Support motor cam 2 (Autodesk Fusion 360 design; units mm, degrees)
Autodesk Fusion 360 part; units mm, degrees
sketch "Support moteur/Cam" plane through (0, 0, 0) normal (0, 0, 1) x (1, 0, 0)
  line L0 (-113.5546, -207.3984) -> (-130.3546, -207.3984)
  line L1 (-130.3546, -207.3984) -> (-135.6849, -205.7263)
  line L2 (-135.6849, -205.7263) -> (-141.4789, -211.9329)
  line L3 (-141.4789, -211.9329) -> (-141.6802, -212.3176)
  line L4 (-141.6802, -212.3176) -> (-141.6802, -223.1)
  line L5 (-113.5528, -238.7984) -> (-130.3528, -238.8003)
  line L6 (-130.3528, -238.8003) -> (-135.6829, -240.4729)
  line L7 (-141.4776, -234.267) -> (-141.679, -233.8823)
  line L8 (-141.679, -233.8823) -> (-141.6802, -223.1)
  line L9 (-135.6829, -240.4729) -> (-141.4776, -234.267)
  circle A0 centre (-136.6035, -217.4087) radius 0.75
  circle A1 centre (-118.6035, -217.4087) radius 0.75
  circle A2 centre (-136.6035, -228.9087) radius 0.75
  circle A3 centre (-118.6035, -228.9087) radius 0.75
  line L10 (-113.5546, -207.3984) -> (-113.5528, -238.7984)
  line L11 (-141.6802, -223.1) -> (-113.5537, -223.0984)
  point P0 (-136.6035, -217.4087)
  point P1 (-118.6035, -217.4087)
  point P2 (-118.6035, -228.9087)
  point P3 (-136.6035, -228.9087)
  dimension "d217" = 16.8
  dimension "d227" = 1.5
  dimension "d228" = 1.5
  dimension "d229" = 1.5
  dimension "d230" = 1.5
  constraint horizontal L0
  constraint vertical L4
  constraint coincident P0 A0.centre
  constraint coincident P1 A1.centre
  constraint coincident P3 A2.centre
  constraint coincident P2 A3.centre
  constraint midpoint L10 L11.end
  constraint perpendicular L10 L11
  measures "d217" distance of L0.start L0.end
  measures "d227" diameter of A0
  measures "d228" diameter of A1
  measures "d229" diameter of A2
  measures "d230" diameter of A3
ref_plane "WorkPlane9" through (0, 0, -10.8) normal (0, 0, 1) x (1, 0, 0)
sketch "Support moteur/Cam2" plane through (0, 0, -10.8) normal (0, 0, 1) x (1, 0, 0)
  line L0 (-113.5546, -236.9984) -> (-130.3974, -237.1164)
  line L1 (-130.3974, -237.1164) -> (-135.6833, -238.6066)
  line L2 (-135.6833, -238.6066) -> (-138.7984, -232.7391)
  line L3 (-138.7984, -223.0984) -> (-138.7984, -232.7391)
  line L4 (-138.7984, -223.0984) -> (-138.7984, -213.4577)
  line L5 (-135.6833, -207.5901) -> (-138.7984, -213.4577)
  line L6 (-130.3974, -209.0804) -> (-135.6833, -207.5901)
  line L7 (-113.5546, -209.1984) -> (-130.3974, -209.0804)
  line L8 (-122.1546, -237.0587) -> (-122.1546, -209.1381)
  line L9 (-113.5546, -209.1984) -> (-113.5546, -236.9984)
  line L10 (-138.7984, -223.0984) -> (-113.5546, -223.0984) construction
  dimension "d221" = 8.6
  constraint coincident L0 L8.start
  constraint coincident L7 L8.end
  constraint vertical L9
  constraint perpendicular L8 L10
  constraint perpendicular L9 L10
  measures "d221" horizontal distance of L0.start L8.start
loft "Loft1" add profiles "Support moteur/Cam2", "Support moteur/Cam" section 1 section 2 contours L0 L1 L2 L3 L4 L10 L11 | L5 L6 L7 L8 L9 L10 L11 | A0 | A1
extrude "Support Moteur/Cam" cut sketch "Support moteur/Cam" against normal blind 8 contours A0 | A1 | A2 | A3
extrude "Extrude10" add sketch "Support moteur/Cam2" against normal blind 29 contours L0 L7 L8 L9
chamfer "Chamfer3" distance 4.9 distance2 28 2 edges at (-117.8546, -209.1683, -39.8) (-117.8546, -237.0285, -39.8) measured on face at (-119.2879, -218.4651, -39.8) measured on face at (-119.2879, -218.4651, -39.8)
fillet "Fillet1" radius 10.5 2 edges at (-117.8546, -232.1284, -39.8) (-117.8546, -214.0684, -39.8)
sketch "Support moteur/Cam3" plane through (-122.1546, 0, 0) normal (-1, 0, 0) x (0, -1, 0)
  ellipse E0 centre (222.8605, -29.3) end of major axis (212.3603, -29.3) minor radius 10.5 (212.5175, -31.11) -> (222.8605, -39.8) ccw
  line L0 (222.8605, -39.8) -> (223.3362, -39.8)
  ellipse E1 centre (223.3362, -29.3) end of major axis (233.8365, -29.3) minor radius 10.5 (223.3362, -39.8) -> (233.6793, -31.11) ccw
  line L1 (233.6793, -31.11) -> (237.0587, -11.8)
  line L2 (237.0587, -11.8) -> (237.0587, -10.8)
  line L3 (237.0587, -10.8) -> (209.1381, -10.8)
  line L4 (209.1381, -10.8) -> (209.1381, -11.8)
  line L5 (209.1381, -11.8) -> (212.5175, -31.11)
  line L6 (223.0984, -10.8) -> (223.0984, -28.5) construction
  line L7 (229.2984, -32.0796) -> (229.2984, -24.9204)
  line L8 (229.2984, -24.9204) -> (223.0984, -21.3409)
  line L9 (223.0984, -21.3409) -> (216.8984, -24.9204)
  line L10 (216.8984, -24.9204) -> (216.8984, -32.0796)
  line L11 (216.8984, -32.0796) -> (223.0984, -35.6591)
  line L12 (223.0984, -35.6591) -> (229.2984, -32.0796)
  circle A0 centre (223.0984, -28.5) radius 1.75
  line L13 (223.0984, -10.8) -> (223.0984, -33.8) construction
  circle A1 centre (223.0984, -33.8) radius 1.6 construction
  circle A2 centre (223.0984, -33.8) radius 3.1 construction
  line L14 (217.8116, -36.9) -> (223.0984, -36.9) construction
  line L15 (221.2654, -36.3) -> (224.9314, -36.3)
  circle A3 centre (223.0984, -33.8) radius 4.1 construction
  point P0 (223.0984, -28.5)
  dimension "d233" = 17.7
  dimension "d235" = 12.4
  dimension "d236" = 3.5
  dimension "d380" = 23
  dimension "d381" = 3.2
  dimension "d382" = 6.2
  dimension "d383" = 0.6
  dimension "d384" = 8.2
  dimension "d395" = 9
  constraint midpoint L3 L6.start
  constraint perpendicular L3 L6
  constraint coincident P0 L6.end
  constraint coincident L6 L8.end
  constraint parallel L6 L13
  constraint coincident L13.end A1.centre
  constraint concentric A1 A2
  constraint horizontal L14
  constraint coincident A2 L14.end
  constraint tangent A2 L14
  constraint coincident A2 L15.start
  constraint coincident A2 L15.end
  constraint parallel L14 L15
  constraint concentric A2 A3
  measures "d233" distance of L6.start P0
  measures "d235" distance of L7 L10
  measures "d236" diameter of A0
  measures "d380" distance of L6.start L13.end
  measures "d381" diameter of A1
  measures "d382" diameter of A2
  measures "d383" distance of L14 L15.start
  measures "d384" diameter of A3
extrude "Extrude12" cut sketch "Support moteur/Cam3" against normal through all contours A0
extrude "Extrude13" cut sketch "Support moteur/Cam3" against normal blind 7.6 contours L7 L8 L9 L10 L11 L12
extrude "Extrude19" [suppressed]
fillet "Fillet2" [suppressed]
equation "Trous_Vis_diam2 = 2.2 mm"
named bodies: "Support moteur/Cam"
